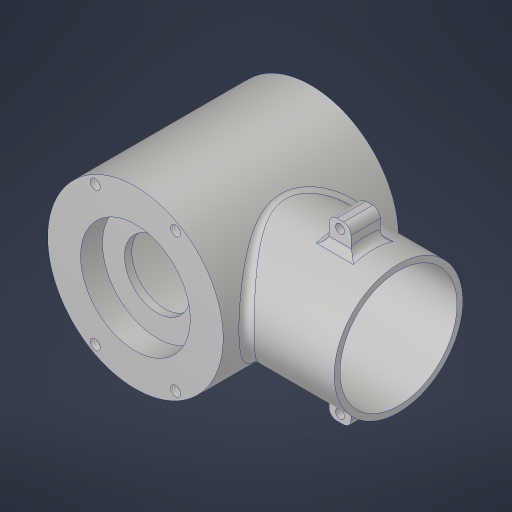
# Autodesk Inventor part: AR-001
Saved by Autodesk Inventor 2023.4 (Build 274418000, 418)
## iProperties
Created: 2025-01-22
Part Number: AR-001
Material: Aluminum 6061
Document SubType Name: Modeling
Designer: jmcintyr
Density: 2.7 g/cm^3
Appearance: Aluminum - Flat
Mass: 424.302 g
Surface Area: 617.506 cm^2
Volume: 157.149 cm^3
Author: jmcintyr
Autodesk Inventor part; units mm, degrees
ref_plane "XZ Plane" through (0, 0, 0) normal (0, 1, 0) x (-1, 0, 0)
sketch "Sketch1" plane through (0, 0, 0) normal (0, 0, 1) x (1, 0, 0)
  circle A0 centre (0, 0) radius 38.1
  dimension "d0" = 76.2
  constraints: 1 centre point, 1 coincident
  measures "d0" diameter of A0
extrude "Extrusion1" add sketch "Sketch1" along normal mid plane 76.2
ref_plane "Work Plane1" through (76.2, 0, 0) normal (1, 0, 0) x (0, 1, 0)
sketch "Sketch2" plane through (76.2, 0, 0) normal (1, 0, 0) x (0, 1, 0)
  circle A0 centre (0, 0) radius 25.4
  circle A1 centre (0, 0) radius 27.94
  dimension "d4" = 50.8
  dimension "d5" = 2.54
  constraints: 2 centre point, 1 coincident
  measures "d4" diameter of A0
  measures "d5" radial gap between concentric circles of A0 A1
extrude "Extrusion2" add sketch "Sketch2" against normal up to next
sketch "Sketch3" plane through (76.2, 0, 0) normal (1, 0, 0) x (0, 1, 0)
  circle A0 centre (0, 0) radius 25.4 projected
extrude "Extrusion3" cut sketch "Sketch3" against normal blind 83.82
sketch "Sketch4" plane through (0, 0, 38.1) normal (0, 0, 1) x (1, 0, 0)
  point P0 (0, 0)
  point P1 (0, 0)
  constraints: 1 coincident
hole "Hole1" at (0, 0, 38.1) direction (0, 0, -1) diameter 28.575 depth 41.275 tip angle 118 counterbore diameter 47.625 counterbore depth 9.525
ref_plane "Work Plane2" through (0, 0, 38.1) normal (0, 0, 1) x (1, 0, 0)
sketch "Sketch6" plane through (0, 0, 38.1) normal (0, 0, 1) x (1, 0, 0)
  line L0 (76.2, 27.94) -> (25.903, 27.94) projected
  line L1 (76.2, -27.94) -> (25.903, -27.94) projected
  circle A0 centre (0, 0) radius 38.1 projected
  line L2 (38.1, 0) -> (76.2, 0) construction
  line L3 (61.9125, 6.35) -> (52.3875, 6.35)
  line L4 (52.3875, 6.35) -> (52.3875, -6.35)
  line L5 (52.3875, -6.35) -> (61.9125, -6.35)
  line L6 (61.9125, -6.35) -> (61.9125, 6.35)
  line L7 (61.9125, 6.35) -> (52.3875, -6.35) construction
  line L8 (52.3875, 6.35) -> (61.9125, -6.35) construction
  point P0 (57.15, 0)
  dimension "d23" = 9.525
  dimension "d24" = 12.7
  constraints: 14 end point, 3 midpoint, 2 horizontal, 2 parallel, 1 perpendicular, 1 point on circle
  measures "d23" distance of L5.end L4.end
  measures "d24" distance of L4.end L3.end
extrude "Extrusion4" add sketch "Sketch6" against normal up to next contours L6 L5 L4 L3
mirror "Mirror1" about plane through (0, 0, 0) normal (0, 0, 1) of "Extrusion4"
ref_plane "Work Plane3" through (-47.625, 0, 0) normal (1, 0, 0) x (0, 1, 0)
sketch "Sketch7" plane through (-47.625, 0, 0) normal (1, 0, 0) x (0, 1, 0)
  line L0 (4.7625, 6.35) -> (-4.7625, 6.35)
  line L1 (-4.7625, 6.35) -> (-4.7625, -6.35)
  line L2 (-4.7625, -6.35) -> (4.7625, -6.35)
  line L3 (4.7625, -6.35) -> (4.7625, 6.35)
  line L4 (4.7625, 6.35) -> (-4.7625, -6.35) construction
  line L5 (-4.7625, 6.35) -> (4.7625, -6.35) construction
  point P0 (0, 0)
  dimension "d28" = 9.525
  dimension "d29" = 12.7
  constraints: 12 end point, 2 midpoint, 2 parallel, 1 horizontal, 1 perpendicular
  measures "d28" distance of L2.end L1.end
  measures "d29" distance of L1.end L0.end
extrude "Extrusion5" add sketch "Sketch7" along normal up to next
fillet "Fillet1" radius 6.604 4 edges at (52.3875, 0, 27.94) (52.3875, 0, -27.94) (61.9125, 0, -27.94) (61.9125, 0, 27.94)
sketch "Sketch8" plane through (0, 0, -38.1) normal (0, 0, -1) x (-1, 0, 0)
  point P0 (0, 0)
  point P1 (0, 0)
  constraints: 1 coincident
hole "Hole2" at (0, 0, -38.1) direction (0, 0, 1) diameter 28.575 end up to surface counterbore diameter 47.625 counterbore depth 9.525
sketch "Sketch9" plane through (0, 0, 0) normal (0, 0, 1) x (1, 0, 0)
  circle A0 centre (0, 0) radius 31.5139
  constraints: 1 centre point, 1 coincident
extrude "Extrusion6" cut sketch "Sketch9" along normal mid plane 50.8
sketch "Sketch10" plane through (0, 0, 38.1) normal (0, 0, 1) x (1, 0, 0)
  circle A0 centre (0, 0) radius 38.1 projected
  circle A1 centre (0, 0) radius 34.8488 construction
  line L0 (17.4625, -30.1625) -> (-17.4625, -30.1625) construction
  line L1 (-17.4625, -30.1625) -> (-17.4625, 30.1625) construction
  line L2 (-17.4625, 30.1625) -> (17.4625, 30.1625) construction
  line L3 (17.4625, 30.1625) -> (17.4625, -30.1625) construction
  line L4 (17.4625, -30.1625) -> (-17.4625, 30.1625) construction
  line L5 (-17.4625, -30.1625) -> (17.4625, 30.1625) construction
  dimension "d43" = 69.6976
  dimension "d44" = 34.925
  dimension "d45" = 60.325
  constraints: 12 end point, 5 coincident, 2 midpoint, 2 parallel, 1 centre point, 1 horizontal, 1 perpendicular
  measures "d43" diameter of A1
  measures "d44" distance of L1.end L2.end
  measures "d45" distance of L0.end L1.end
hole "Hole3" at (-17.4625, 30.1625, 38.1) at (17.4625, 30.1625, 38.1) at (17.4625, -30.1625, 38.1) at (-17.4625, -30.1625, 38.1) direction (0, 0, -1) diameter 4.3434 end through all thread size "12-24 UNC" class "2B" standard "ANSI Unified Screw Threads"
fillet "Fillet2" radius 3.302 12 edges at (31.6413, 21.2236, 18.1715) (31.6407, -21.2244, 18.1706) (31.6413, -21.2236, -18.1715) (31.6413, 21.2235, -18.1716) (57.15, 6.35, 27.2088) (57.15, -6.35, 27.2088) (52.3875, 0, -38.1) (61.9125, 0, -38.1) (61.9125, 0, 38.1) (52.3875, 0, 38.1) (57.15, 6.35, -27.2088) (57.15, -6.35, -27.2088)
sketch "Sketch11" plane through (55.6895, 6.35, 38.1) normal (0, 1, 0) x (1, 0, 0)
  line L0 (-93.2566, 0) -> (-93.2566, 76.2) projected
  line L1 (-78.6397, 0) -> (-93.2566, 0) projected
  line L2 (-78.6397, 9.525) -> (-78.6397, 0) projected
  line L3 (-68.4883, 9.525) -> (-78.6397, 9.525) projected
  line L4 (-68.4883, 12.7) -> (-68.4883, 9.525) projected
  line L5 (-86.557, 12.7) -> (-68.4883, 12.7) projected
  line L6 (-86.557, 63.5) -> (-86.557, 12.7) projected
  line L7 (-68.4883, 63.5) -> (-86.557, 63.5) projected
  line L8 (-68.4883, 66.675) -> (-68.4883, 63.5) projected
  line L9 (-78.6397, 66.675) -> (-68.4883, 66.675) projected
  line L10 (-78.6397, 76.2) -> (-78.6397, 66.675) projected
  line L11 (-93.2566, 76.2) -> (-78.6397, 76.2) projected
  line L12 (-14.9009, 65.3088) -> (-9.906, 65.3088) projected
  line L13 (12.827, 65.3088) -> (20.5105, 65.3088) projected
  line L14 (20.5105, 13.5066) -> (20.5105, 10.8912) projected
  line L15 (-24.822, 13.5066) -> (20.5105, 13.5066) projected
  line L16 (-24.822, 62.6934) -> (-24.822, 63.5) projected
  line L17 (-24.822, 63.5) -> (-42.8907, 63.5) projected
  line L18 (-42.8907, 63.5) -> (-42.8907, 66.675) projected
  line L19 (-42.8907, 66.675) -> (-32.7393, 66.675) projected
  line L20 (-32.7393, 66.675) -> (-32.7393, 76.2) projected
  line L21 (-32.7393, 76.2) -> (-18.1224, 76.2) projected
  line L22 (-18.1224, 76.2) -> (-18.1224, 68.5704) projected
  line L23 (-3.302, 72.0553) -> (-3.302, 72.898) projected
  arc A0 (0, 76.2) -> (-3.302, 72.898) centre (0, 72.898) ccw projected
  line L24 (0, 76.2) -> (2.921, 76.2) projected
  arc A1 (6.223, 72.898) -> (2.921, 76.2) centre (2.921, 72.898) ccw projected
  line L25 (6.223, 72.898) -> (6.223, 72.0553) projected
  line L26 (20.5105, 10.8912) -> (12.827, 10.8912) projected
  line L27 (7.6975, 8.3863) -> (-4.7765, 8.3863) projected
  line L28 (-3.302, 3.302) -> (-3.302, 4.1447) projected
  arc A2 (-3.302, 3.302) -> (0, 0) centre (0, 3.302) ccw projected
  line L29 (2.921, 0) -> (0, 0) projected
  arc A3 (2.921, 0) -> (6.223, 3.302) centre (2.921, 3.302) ccw projected
  line L30 (6.223, 4.1447) -> (6.223, 3.302) projected
  line L31 (20.5105, 65.3088) -> (20.5105, 62.6934) projected
  line L32 (20.5105, 62.6934) -> (-24.822, 62.6934) projected
  line L33 (-42.8907, 12.7) -> (-24.822, 12.7) projected
  line L34 (-42.8907, 9.525) -> (-42.8907, 12.7) projected
  line L35 (-32.7393, 9.525) -> (-42.8907, 9.525) projected
  line L36 (-32.7393, 0) -> (-32.7393, 9.525) projected
  line L37 (-18.1224, 0) -> (-32.7393, 0) projected
  line L38 (-9.906, 10.8912) -> (-14.9009, 10.8912) projected
  line L39 (0, 72.898) -> (2.921, 72.898) construction
  line L40 (0, 3.302) -> (2.921, 3.302) construction
  line L41 (-4.7765, 67.8137) -> (7.6975, 67.8137) projected
  line L42 (-24.822, 12.7) -> (-24.822, 13.5066) projected
  line L43 (-18.1224, 7.6296) -> (-18.1224, 0) projected
  point P0 (-55.6895, 38.1)
  point P1 (-100.0125, 25.527)
  point P2 (-100.0125, 50.673)
  point P3 (1.4605, 3.302)
  point P4 (1.4605, 72.898)
  point P5 (-100.0125, 50.673)
  point P6 (-100.0125, 25.527)
  constraints: 4 end point, 2 coincident, 2 horizontal, 2 midpoint, 10 other
hole "Hole4" at (57.15, 6.35, 34.798) at (-44.323, 6.35, 12.573) at (57.15, 6.35, -34.798) direction (0, -1, 0) diameter 3.9624 end through all thread size "10-32 UNF" class "2B" standard "ANSI Unified Screw Threads"
pattern_circular "Circular Pattern1" count 2 over 90 about axis through (76.2, 0, 0) along (-1, 0, 0) of "Extrusion4", "Mirror1", "Hole4"
fillet "Fillet3" radius 3.302 14 edges at (61.9125, 27.7566, -3.196) (61.9125, 27.7566, 3.196) (57.15, 27.2088, 6.35) (61.9125, 38.1, 0) (52.3875, 38.1, 0) (52.3875, 27.7566, -3.196) (52.3875, 27.7566, 3.196) (57.15, 27.2088, -6.35) (61.9125, -27.94, 0) (57.15, -27.2088, 6.35) (52.3875, -27.94, 0) (57.15, -27.2088, -6.35) (61.9125, -38.1, 0) (52.3875, -38.1, 0)
sketch "Sketch12" plane through (76.2, 0, 0) normal (1, 0, 0) x (0, 0, -1)
  circle A0 centre (0, 0) radius 27.94 construction
  circle A1 centre (0, 0) radius 25.4 construction
  circle A2 centre (0, 0) radius 50.8 construction
  circle A3 centre (0, 0) radius 27.94 construction
  arc A4 (24.8868, -12.7) -> (24.8868, 12.7) centre (0, 0) ccw
  arc A5 (49.1869, -12.7) -> (49.1869, 12.7) centre (0, 0) ccw
  arc A6 (-49.1869, 12.7) -> (-49.1869, -12.7) centre (0, 0) ccw
  arc A7 (-24.8868, 12.7) -> (-24.8868, -12.7) centre (0, 0) ccw
  line L0 (49.1869, -12.7) -> (24.8868, -12.7)
  line L1 (-24.8868, -12.7) -> (-49.1869, -12.7)
  line L2 (-49.1869, 12.7) -> (-24.8868, 12.7)
  line L3 (-38.1, -23.8125) -> (-38.1, 23.8125) construction
  line L4 (49.1869, 12.7) -> (24.8868, 12.7)
  line L5 (37.0369, -12.7) -> (37.0369, 12.7) construction
  line L6 (-37.0369, 12.7) -> (-37.0369, -12.7) construction
  point P0 (37.0369, 0)
  point P1 (-37.0369, 0)
  dimension "d64" = 25.4
  dimension "d65" = 25.4
  dimension "d66" = 101.6
  constraints: 16 point on circle, 12 end point, 6 midpoint, 5 centre point, 5 coincident, 3 concentric, 3 horizontal, 3 perpendicular, 2 horizontal alignment
  measures "d64" distance between parallel lines of L4 L0
  measures "d65" distance between parallel lines of L1 L2
  measures "d66" diameter of A2
extrude "Extrusion7" cut sketch "Sketch12" against normal blind 31.75
fillet "Fillet4" radius 3.302 6 edges at (-38.1, 0, 6.35) (-37.8012, -4.7625, 0) (-38.1, 0, -6.35) (-37.8012, 4.7625, 0) (-47.625, -4.7625, 0) (-47.625, 4.7625, 0)
sketch "Sketch13" plane through (-47.625, -1.4605, -6.35) normal (0, 0, -1) x (-1, 0, 0)
  circle A0 centre (-104.775, 36.2585) radius 1.9812 construction
  circle A1 centre (-104.775, -33.3375) radius 1.9812 construction
  circle A2 centre (-65.0875, -28.702) radius 2.1717 construction
  circle A3 centre (-30.1625, 31.623) radius 2.1717 construction
  circle A4 centre (-65.0875, 31.623) radius 2.1717 construction
  circle A5 centre (-30.1625, -28.702) radius 2.1717 construction
  arc A6 (-67.33, -23.1329) -> (-67.33, 26.0539) centre (-47.625, 1.4605) ccw construction
  line L0 (-67.33, 26.0539) -> (-123.825, 26.0539) construction
  line L1 (-123.825, 26.0539) -> (-123.825, 28.6693) construction
  line L2 (-123.825, 28.6693) -> (-112.8395, 28.6693) construction
  line L3 (-109.6508, 31.1742) -> (-99.8992, 31.1742) construction
  line L4 (-96.7105, 28.6693) -> (-75.7049, 28.6693) construction
  arc A7 (-10.2548, 8.8818) -> (-73.2994, 29.6107) centre (-47.625, 1.4605) ccw construction
  arc A8 (-10.2548, 8.8818) -> (-7.016, 6.223) centre (-7.016, 9.525) ccw construction
  line L5 (-7.016, 6.223) -> (-6.4978, 6.223) construction
  arc A9 (-6.4978, -3.302) -> (-6.4978, 6.223) centre (-47.625, 1.4605) ccw construction
  line L6 (-3.302, -3.302) -> (-6.4978, -3.302) construction
  arc A10 (-3.302, -3.302) -> (0, 0) centre (-3.302, 0) ccw construction
  line L7 (0, 2.921) -> (0, 0) construction
  arc A11 (0, 2.921) -> (-3.302, 6.223) centre (-3.302, 2.921) ccw construction
  line L8 (-6.4978, 6.223) -> (-3.302, 6.223) construction
  line L9 (-123.825, -23.1329) -> (-67.33, -23.1329) construction
  line L10 (-123.825, -25.7483) -> (-123.825, -23.1329) construction
  line L11 (-112.8395, -25.7483) -> (-123.825, -25.7483) construction
  line L12 (-99.8992, -28.2532) -> (-109.6508, -28.2532) construction
  line L13 (-100.0125, -29.1294) -> (-100.0125, -33.3375) construction
  arc A12 (-103.3145, -36.6395) -> (-100.0125, -33.3375) centre (-103.3145, -33.3375) ccw construction
  line L14 (-103.3145, -36.6395) -> (-106.2355, -36.6395) construction
  arc A13 (-109.5375, -33.3375) -> (-106.2355, -36.6395) centre (-106.2355, -33.3375) ccw construction
  line L15 (-109.5375, -33.3375) -> (-109.5375, -29.1294) construction
  line L16 (-109.5375, 32.0504) -> (-109.5375, 36.2585) construction
  arc A14 (-106.2355, 39.5605) -> (-109.5375, 36.2585) centre (-106.2355, 36.2585) ccw construction
  line L17 (-106.2355, 39.5605) -> (-103.3145, 39.5605) construction
  arc A15 (-100.0125, 36.2585) -> (-103.3145, 39.5605) centre (-103.3145, 36.2585) ccw construction
  line L18 (-100.0125, 36.2585) -> (-100.0125, 32.0504) construction
  line L19 (-6.4978, -3.302) -> (-7.016, -3.302) construction
  arc A16 (-7.016, -3.302) -> (-10.2548, -5.9608) centre (-7.016, -6.604) ccw construction
  arc A17 (-73.2994, -26.6897) -> (-10.2548, -5.9608) centre (-47.625, 1.4605) ccw construction
  line L20 (-75.7049, -25.7483) -> (-96.7105, -25.7483) construction
  line L21 (-3.302, 0) -> (-3.302, 2.921) construction
  point P0 (-3.302, 1.4605)
  constraints: 2 end point, 1 midpoint, 1 vertical, 10 other
hole "Hole5" at (-44.323, 0, -6.35) direction (0, 0, 1) diameter 3.9624 end through all thread size "10-32 UNF" class "2B" standard "ANSI Unified Screw Threads"
body "Solid1"
